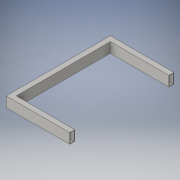
# Autodesk Inventor part: MiddleNarrowFrameMoutingForMotors
Saved by Autodesk Inventor 2016 SP1 (Build 200210100, 210)
## iProperties
Created: 2016-01-24
Part Number: MiddleNarrowFrameMoutingForMotors
Material: Generic
Document SubType Name: Modeling
Designer: steele
Density: 1 g/cm^3
Appearance: Default
Author: steele
Autodesk Inventor part; units mm, degrees
ref_plane "XZ Plane" through (0, 0, 0) normal (0, 1, 0) x (-1, 0, 0)
ref_plane "XY Plane" through (0, 0, 0) normal (0, 0, 1) x (1, 0, 0)
sketch "Sketch10" plane through (0, 0, 0) normal (0, 1, 0) x (-1, 0, 0)
  line L0 (0, 0) -> (0, 247.65)
  line L1 (0, 247.65) -> (-304.8, 247.65)
  line L2 (0, 0) -> (-304.8, 0) construction
  line L3 (0, 0) -> (0, -247.65)
  line L4 (0, -247.65) -> (-304.8, -247.65)
  dimension "d31" = 247.65
  dimension "d32" = 304.8
  constraints: 10 end point, 2 symmetric about line, 1 horizontal, 1 perpendicular, 1 vertical
  measures "d31" distance of L0.start L0.end
  measures "d32" distance of L0.end L1.end
ref_plane "Work Plane2" through (304.8, 0, 0) normal (1, 0, 0) x (0, 1, 0)
sketch "Sketch11" plane through (304.8, 0, 0) normal (1, 0, 0) x (0, 1, 0)
  line L0 (-25.4, 260.35) -> (-25.4, 234.95)
  line L1 (-25.4, 234.95) -> (25.4, 234.95)
  line L2 (25.4, 234.95) -> (25.4, 260.35)
  line L3 (25.4, 260.35) -> (-25.4, 260.35)
  line L4 (-25.4, 260.35) -> (25.4, 234.95) construction
  line L5 (-25.4, 234.95) -> (25.4, 260.35) construction
  line L6 (-22.225, 257.175) -> (-22.225, 238.125)
  line L7 (-22.225, 238.125) -> (22.225, 238.125)
  line L8 (22.225, 238.125) -> (22.225, 257.175)
  line L9 (22.225, 257.175) -> (-22.225, 257.175)
  line L10 (-22.225, 257.175) -> (22.225, 238.125) construction
  line L11 (-22.225, 238.125) -> (22.225, 257.175) construction
  point P0 (0, 0)
  point P1 (0, 247.65)
  dimension "d34" = 247.65
  dimension "d35" = 25.4
  dimension "d36" = 50.8
  dimension "d37" = 3.175
  dimension "d38" = 3.175
  constraints: 24 end point, 4 midpoint, 4 parallel, 2 perpendicular, 2 vertical
  measures "d34" distance of point (0, 0) point (0, 247.65)
  measures "d35" distance of L1.end L2.end
  measures "d36" distance of L2.end L0.start
  measures "d37" distance between parallel lines of L3 L9
  measures "d38" distance between parallel lines of L0 L6
sweep "Sweep5" add profiles "Sketch11" path "Sketch10" path curves L1 L0 L3 L4
equation "\"d31\" = halfOfWidth"
equation "\"d32\" = length"
equation "\"d34\" = halfOfWidth"
equation "\"d35\" = tubingWidth"
equation "\"d36\" = tubingHeight"
equation "\"d37\" = tubeThickness"
equation "\"d38\" = tubeThickness"
equation "\"halfOfWidth\" = 247.65"
equation "\"length\" = 304.8"
equation "\"height\" = 241.3"
equation "\"tubingWidth\" = 25.4"
equation "\"tubingHeight\" = 50.8"
equation "\"tubeThickness\" = 3.175"
equation "\"d33\" = length"
equation "\"width\" = 508"
body "Solid5"
